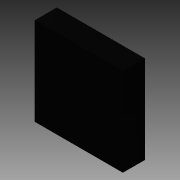
# Autodesk Inventor part: Si7021
Saved by Autodesk Inventor 2013 (Build 170138000, 138)
## iProperties
Created: 2015-06-30
Part Number: Si7021
Material: Ogólny
Document SubType Name: Modeling
Designer: terg
Density: 1 g/cm^3
Author: terg
Autodesk Inventor part; units mm, degrees
ref_plane "YZ Plane" through (0, 0, 0) normal (1, 0, 0) x (0, 1, 0)
ref_plane "XZ Plane" through (0, 0, 0) normal (0, 1, 0) x (-1, 0, 0)
ref_plane "XY Plane" through (0, 0, 0) normal (0, 0, 1) x (1, 0, 0)
sketch "Szkic1" plane through (0, 0, 0) normal (0, 1, 0) x (-1, 0, 0)
  line L0 (0, 0) -> (3, 0)
  line L1 (3, 0) -> (3, 3)
  line L2 (3, 3) -> (0, 3)
  line L3 (0, 3) -> (0, 0)
  dimension "d0" = 3
  dimension "d1" = 3
  constraints: 8 end point, 2 parallel, 1 horizontal, 1 perpendicular
  measures "d0" distance of L2.end L1.end
  measures "d1" distance of L1.end L0.end
extrude "Wyciągnięcie proste1" add sketch "Szkic1" along normal blind 0.75
sketch "Szkic2" plane through (0, 0.75, 0) normal (0, 1, 0) x (1, 0, 0)
  line L0 (0, 0) -> (-3, 0) projected
  line L1 (-3, 0) -> (-3, -3) projected
  line L2 (-3, -3) -> (0, -3) projected
  line L3 (0, -3) -> (0, 0) projected
  line L4 (-1.8629, -0.1) -> (-0.6, -0.1)
  line L5 (-0.1, -0.6) -> (-0.1, -2.4)
  line L6 (-0.6, -2.9) -> (-2.4, -2.9)
  line L7 (-2.9, -2.4) -> (-2.9, -1.1371)
  line L8 (-2.7536, -0.7836) -> (-2.2164, -0.2464)
  arc A0 (-2.9, -2.4) -> (-2.4, -2.9) centre (-2.4, -2.4) ccw
  arc A1 (-0.6, -2.9) -> (-0.1, -2.4) centre (-0.6, -2.4) ccw
  arc A2 (-0.1, -0.6) -> (-0.6, -0.1) centre (-0.6, -0.6) ccw
  arc A3 (-2.7536, -0.7836) -> (-2.9, -1.1371) centre (-2.4, -1.1371) ccw
  arc A4 (-1.8629, -0.1) -> (-2.2164, -0.2464) centre (-1.8629, -0.6) ccw
  point P0 (-2.07, -0.1)
  point P1 (-0.1, -2.9)
  point P2 (-0.1, -0.1)
  point P3 (-2.9, -2.9)
  point P4 (-2.9, -0.93)
  dimension "d4" = 2.8
  dimension "d5" = 2.8
  dimension "d6" = 0.1
  dimension "d7" = 0.1
  dimension "d8" = 0.1
  dimension "d9" = 0.1
  dimension "d10" = 0.83
  dimension "d11" = 0.83
  dimension "d12" = 0.5
  dimension "d13" = 0.5
  constraints: 10 end point, 10 point on circle, 10 point on line, 10 tangent, 5 centre point, 3 equal radius, 2 parallel, 1 horizontal, 1 perpendicular
  measures "d4" distance of point (-0.1, -2.9) point (-2.9, -2.9)
  measures "d5" distance of point (-0.1, -0.1) point (-0.1, -2.9)
  measures "d6" distance between parallel lines of L1 L7
  measures "d7" distance between parallel lines of L3 L5
  measures "d8" distance between parallel lines of L0 L4
  measures "d9" distance between parallel lines of L2 L6
  measures "d10" distance from line of point (-2.9, -0.93) L4
  measures "d11" distance from line of point (-2.07, -0.1) L7
  measures "d12" radius of A0
  measures "d13" radius of A1
extrude "Wyciągnięcie proste2" add sketch "Szkic2" along normal blind 0.01 contours L4 A2 L5 A1 L6 A0 L7 A3 L8 A4
sketch "Szkic3" plane through (0, 0.75, 0) normal (0, 1, 0) x (1, 0, 0)
  line L0 (0, 0) -> (-3, 0) projected
  line L1 (-3, 0) -> (-3, -3) projected
  point P0 (-2.6, -0.4)
  dimension "d16" = 0.4
  dimension "d17" = 0.4
  measures "d16" distance from line of L0 point (-2.6, -0.4)
  measures "d17" distance from line of L1 point (-2.6, -0.4)
hole "Otwór1" at (-2.6, 0.75, 0.4) direction (0, -1, 0) diameter 0.3 depth 0.1
equation "\"d6\" = d7"
equation "\"d8\" = d9"
